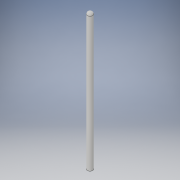
# Autodesk Inventor part: Part9
Saved by Autodesk Inventor 2019 (Build 230136000, 136)
## iProperties
Created: 2019-01-18
Part Number: Part9
Material: Generic
Document SubType Name: Modeling
Designer: mar22
Density: 1 g/cm^3
Appearance: Default
Author: mar22
Autodesk Inventor part; units mm, degrees
ref_plane "YZ Plane" through (0, 0, 0) normal (1, 0, 0) x (0, 1, 0)
ref_plane "XZ Plane" through (0, 0, 0) normal (0, 1, 0) x (-1, 0, 0)
ref_plane "XY Plane" through (0, 0, 0) normal (0, 0, 1) x (1, 0, 0)
sketch "Sketch1" plane through (0, 0, 0) normal (1, 0, 0) x (0, 1, 0)
  line L0 (317.5, -12.7) -> (-317.5, -12.7)
  line L1 (-317.5, -12.7) -> (-317.5, 0)
  arc A0 (317.5, -12.7) -> (330.2, 0) centre (317.5, 0) ccw
  line L2 (330.2, 0) -> (-317.5, 0)
  line L3 (386.259, 0) -> (-534.3178, 0)
  point P0 (0, 0)
  constraints: 8 end point, 2 horizontal, 2 point on circle, 1 centre point
revolve "Revolution1" add sketch "Sketch1" angle 360 about axis through (0, 386.259, 0) along (0, -1, 0)
body "Solid1"
